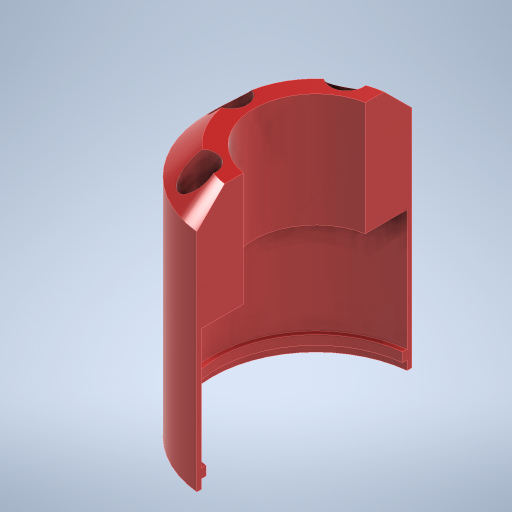
# Autodesk Inventor part: Clamp
Saved by Autodesk Inventor 2024 (Build 280153000, 153)
## iProperties
Created: 2023-09-22
Part Number: Clamp
Material: Brass, Soft Yellow, Welded
Document SubType Name: Modeling
Designer: schanen
Density: 8.5 g/cm^3
Appearance: Red
Author: schanen
Autodesk Inventor part; units mm, degrees
ref_plane "YZ Plane" through (0, 0, 0) normal (1, 0, 0) x (0, 1, 0)
ref_plane "XZ Plane" through (0, 0, 0) normal (0, 1, 0) x (-1, 0, 0)
ref_plane "XY Plane" through (0, 0, 0) normal (0, 0, 1) x (1, 0, 0)
sketch "Sketch1" plane through (0, 0, 0) normal (0, 0, 1) x (1, 0, 0)
  line L0 (-13.5, 30.3) -> (-13.5, 55)
  line L1 (-13.5, 55) -> (-17.5, 55)
  line L2 (-17.5, 55) -> (-23.5, 49)
  line L3 (-23.5, 49) -> (-23.5, 0)
  line L4 (-23.5, 0) -> (-22.5, 0)
  line L5 (-22.5, 0) -> (-22.5, 2)
  line L6 (-22.5, 2) -> (-21.5, 2)
  line L7 (-21.5, 2) -> (-21.5, 4)
  line L8 (-21.5, 4) -> (-22.5, 4)
  line L9 (-22.5, 4) -> (-22.5, 30.3)
  line L10 (-22.5, 30.3) -> (-13.5, 30.3)
  line L11 (0, -11) -> (0, 66) projected
  point P0 (0, 0)
  point P1 (-23, 0)
  point P2 (-21.5, 3)
  dimension "d5" = 24.7
  dimension "d6" = 2
  dimension "d7" = 2
  dimension "d8" = 45
  dimension "d9" = 13.5
  dimension "d10" = 23.5
  dimension "d11" = 49
  dimension "d12" = 1
  dimension "d13" = 2
  dimension "d24" = 55
  constraints: 22 end point, 7 perpendicular, 2 midpoint, 2 point on line, 1 horizontal alignment, 1 parallel, 1 vertical
  measures "d5" distance of L0.start L0.end
  measures "d6" distance of L6.end L7.end
  measures "d7" distance of L4.end L5.end
  measures "d8" angle of L1 L2
  measures "d9" distance between parallel lines of L11 L0
  measures "d10" distance between parallel lines of L11 L3
  measures "d11" distance of L2.end L3.end
  measures "d12" distance of L5.end L6.end
  measures "d13" distance from line of L3 point (-21.5, 3)
  measures "d24" distance from line of L4.end L1
revolve "Revolution1" add sketch "Sketch1" angle 360 about axis through (0, -10, 0) along (0, 1, 0)
sketch "Sketch2" plane through (0, 55, 0) normal (0, 1, 0) x (1, 0, 0)
  line L0 (23.5, -23.5) -> (-2.5, -23.5)
  line L1 (-2.5, -23.5) -> (-2.5, 23.5)
  line L2 (-2.5, 23.5) -> (23.5, 23.5)
  line L3 (23.5, 23.5) -> (23.5, -23.5)
  circle A0 centre (0, 0) radius 23.5 projected
  point P0 (-2.5, 0)
  point P1 (23.5, 0)
  point P2 (0, -23.5)
  point P3 (0, 23.5)
  point P4 (-2.5, 23.3666)
  point P5 (-2.5, -23.3666)
  dimension "d1" = 2.5
  constraints: 8 end point, 3 tangent, 2 midpoint, 2 parallel, 1 horizontal, 1 perpendicular
  measures "d1" distance of point (-2.5, 0) point (0, 0)
extrude "Extrusion1" cut sketch "Sketch2" against normal through all contours L0 A0 L3 | A0 L1 | A0 L2 L3 picked at (6.1667, 0)
sketch "Sketch3" plane through (0, 55, 0) normal (0, 1, 0) x (1, 0, 0)
  circle A0 centre (0, 0) radius 18.5 construction
  point P0 (-18.5, 0)
  point P1 (-9.25, 16.0215)
  point P2 (-9.25, -16.0215)
  dimension "d14" = 37
  dimension "d15" = 60
  dimension "d16" = 60
  constraints: 3 point on circle, 1 centre point, 1 coincident, 1 horizontal alignment
  measures "d14" diameter of A0
hole "Hole1" at (-18.5, 55, 0) at (-9.25, 55, -16.0215) at (-9.25, 55, 16.0215) direction (0, -1, 0) diameter 3.242 end through all counterbore diameter 7.2 counterbore depth 14.2 thread size "M4x0.7" class "6H" standard "ANSI Metric M Profile"
body "Solid1"
